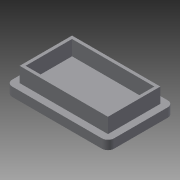
# Autodesk Inventor part: Tapa
Saved by Autodesk Inventor 2013 (Build 170138000, 138)
## iProperties
Created: 2014-07-03
Part Number: Tapa
Material: Genérico
Document SubType Name: Chapa
Designer: Administrador
Density: 1 g/cm^3
Sheet Metal Rule: Por defecto_mm
Author: Administrador
Autodesk Inventor part; units mm, degrees
ref_plane "YZ Plane" through (0, 0, 0) normal (1, 0, 0) x (0, 1, 0)
ref_plane "XZ Plane" through (0, 0, 0) normal (0, 1, 0) x (-1, 0, 0)
ref_plane "XY Plane" through (0, 0, 0) normal (0, 0, 1) x (1, 0, 0)
sketch "Boceto1" plane through (0, 0, 0) normal (0, 0, 1) x (1, 0, 0)
  line L0 (-7.2671, 8.5953) -> (26.7329, 8.5953)
  line L1 (26.7329, 8.5953) -> (26.7329, -13.4047)
  line L2 (26.7329, -13.4047) -> (-7.2671, -13.4047)
  line L3 (-7.2671, -13.4047) -> (-7.2671, 8.5953)
  point P0 (0, 0)
  dimension "d0" = 34
  dimension "d1" = 22
  constraints: 8 end point, 2 parallel, 1 horizontal, 1 perpendicular
  measures "d0" distance of L1.end L2.end
  measures "d1" distance of L0.end L1.end
extrude "Extrusión1" add sketch "Boceto1" along normal blind 3
sketch "Boceto2" plane through (0, 0, 3) normal (0, 0, 1) x (1, 0, 0)
  line L0 (-7.2671, 8.5953) -> (26.7329, -13.4047) construction
  line L1 (26.7329, 8.5953) -> (-7.2671, -13.4047) construction
  line L2 (-5.0171, 6.3453) -> (24.4829, 6.3453)
  line L3 (24.4829, 6.3453) -> (24.4829, -11.1547)
  line L4 (24.4829, -11.1547) -> (-5.0171, -11.1547)
  line L5 (-5.0171, -11.1547) -> (-5.0171, 6.3453)
  line L6 (-5.0171, 6.3453) -> (24.4829, -11.1547) construction
  line L7 (-5.0171, -11.1547) -> (24.4829, 6.3453) construction
  line L8 (-4.0171, 5.3453) -> (23.4829, 5.3453)
  line L9 (23.4829, 5.3453) -> (23.4829, -10.1547)
  line L10 (23.4829, -10.1547) -> (-4.0171, -10.1547)
  line L11 (-4.0171, -10.1547) -> (-4.0171, 5.3453)
  line L12 (-4.0171, 5.3453) -> (23.4829, -10.1547) construction
  line L13 (23.4829, 5.3453) -> (-4.0171, -10.1547) construction
  point P0 (0, 0)
  point P1 (9.7329, -2.4047)
  dimension "d4" = 29.5
  dimension "d5" = 17.5
  dimension "d6" = 27.5
  dimension "d7" = 15.5
  constraints: 28 end point, 4 parallel, 3 midpoint, 2 horizontal, 2 perpendicular
  measures "d4" distance of L3.end L4.end
  measures "d5" distance of L2.end L3.end
  measures "d6" distance of L9.end L10.end
  measures "d7" distance of L8.end L9.end
extrude "Extrusión2" add sketch "Boceto2" along normal blind 5
fillet "Empalme1" radius 2 4 edges at (26.7329, 8.5953, 1.5) (-7.2671, 8.5953, 1.5) (26.7329, -13.4047, 1.5) (-7.2671, -13.4047, 1.5)
equation "\"Radio_pliegue\" = Grosor"
equation "\"Anchura_desahogo_plegado\" = Grosor"
equation "\"Profundidad_desahogo_plegado\" = 0.5 * Grosor"
equation "\"Tamaño_destalonado\" = 4 * Grosor"
equation "\"Remanente_mínimo\" = 2 * Grosor"
equation "\"Radiodetransición\" = Radio_pliegue"
equation "\"Tamaño_de_radio_de_Jacobi\" = Radio_pliegue"
equation "\"TamañoSeparación\" = Grosor"
equation "\"Grosor\" = 0.5"
